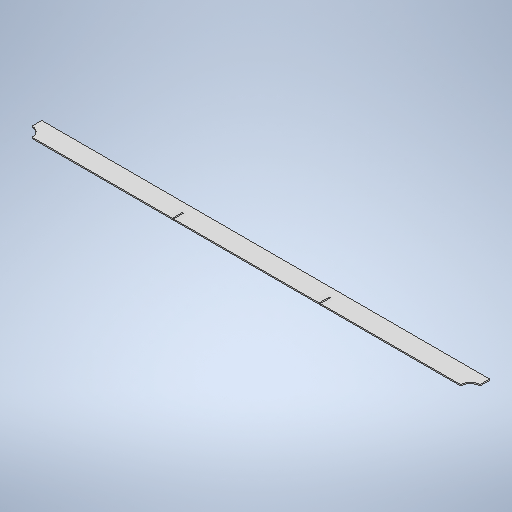
# Autodesk Inventor part: MSC 0563 rib cone
Saved by Autodesk Inventor 2025 (Build 290162010, 162A)
## iProperties
Created: 2024-06-26
Part Number: MSC 0563 rib cone
Material: Stainless Steel
Document SubType Name: Sheet Metal
Designer: pokla
Density: 8 g/cm^3
Sheet Metal Rule: AISI304 3mm Die 32
Appearance: Default
Author: pokla
Autodesk Inventor part; units mm, degrees
ref_plane "YZ Plane" through (0, 0, 0) normal (1, 0, 0) x (0, 1, 0)
ref_plane "XZ Plane" through (0, 0, 0) normal (0, 1, 0) x (-1, 0, 0)
ref_plane "XY Plane" through (0, 0, 0) normal (0, 0, 1) x (1, 0, 0)
sketch "Sketch1" plane through (0, 0, 0) normal (0, 0, 1) x (1, 0, 0)
  line L0 (-580, 50) -> (580, 50)
  line L1 (580, 50) -> (580, 0)
  line L2 (580, 0) -> (-580, 0)
  line L3 (-580, 0) -> (-580, 50)
  circle A0 centre (-580, 0) radius 25
  circle A1 centre (580, 0) radius 25
  point P0 (0, 0)
  point P1 (0, 0)
  point P2 (-580, 25)
  point P3 (-555, 0)
  point P4 (555, 0)
  point P5 (580, 25)
  dimension "d16" = 50
  dimension "d17" = 1160
  dimension "d18" = 50
  dimension "d19" = 50
  measures "d16" distance of L0.end L1.end
  measures "d17" distance of L0.start L0.end
  measures "d18" diameter of A0
  measures "d19" diameter of A1
extrude "Plate2" add sketch "Sketch1" against normal blind 3 contours L0 L1 A1 L2 A0 L3
sketch "Sketch2" plane through (0, 0, 0) normal (0, 0, 1) x (1, 0, 0)
  line L0 (-555, 0) -> (555, 0) projected
  line L1 (190, 0) -> (190, 50) construction
  line L2 (580, 50) -> (-580, 50) projected
  line L3 (188.5, 26) -> (191.5, 26)
  line L4 (191.5, 26) -> (191.5, 0)
  line L5 (191.5, 0) -> (188.5, 0)
  line L6 (188.5, 0) -> (188.5, 26)
  line L7 (-190, 50) -> (-190, 0) construction
  line L8 (-191.5, 26) -> (-188.5, 26)
  line L9 (-188.5, 26) -> (-188.5, 0)
  line L10 (-188.5, 0) -> (-191.5, 0)
  line L11 (-191.5, 0) -> (-191.5, 26)
  point P0 (0, 0)
  point P1 (0, 0)
  point P2 (191.5, 0)
  point P3 (0, 0)
  point P4 (-188.5, 0)
  dimension "d21" = 190
  dimension "d22" = 3
  dimension "d23" = 26
  dimension "d29" = 190
  dimension "d30" = 3
  dimension "d31" = 26
  constraints: 20 end point, 4 midpoint, 4 parallel, 4 point on line, 3 perpendicular, 2 horizontal, 1 vertical
  measures "d21" distance from line of point (0, 0) L1
  measures "d22" distance of L4.end L5.end
  measures "d23" distance of L3.end L4.end
  measures "d29" distance from line of point (0, 0) L7
  measures "d30" distance of L9.end L10.end
  measures "d31" distance of L8.end L9.end
extrude "Extrusion1" cut sketch "Sketch2" against normal through all
equation "\"d22\" = Thickness"
equation "\"d29\" = d21"
equation "\"d30\" = Thickness"
equation "\"d31\" = d23"
equation "\"d20\" = Thickness"
equation "\"BendReliefWidth\" = Thickness"
equation "\"BendReliefDepth\" = 0.5 * Thickness"
equation "\"CornerReliefSize\" = 4 * Thickness"
equation "\"MinimumRemnant\" = 2 * Thickness"
equation "\"TransitionRadius\" = BendRadius"
equation "\"JacobiRadiusSize\" = BendRadius"
equation "\"GapSize\" = Thickness"
equation "\"Thickness\" = 3"
equation "\"BendRadius\" = 5"
body "Solid2"
